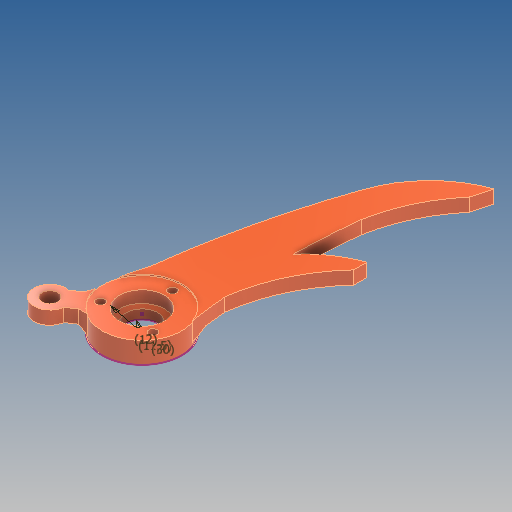
# Autodesk Inventor part: 01-03-01 Zange links nue
Saved by Autodesk Inventor 2026.2 (Build 302298000, 298)
## iProperties
Created: 2025-12-11
Part Number: 01-03-01 Zange links nue
Material: Phenolharz
Document SubType Name: Modeling
Designer: Schally
Density: 1.38 g/cm^3
Appearance: Glatt - Hellorange
Author: Schally
Autodesk Inventor part; units mm, degrees
sketch "Skizze10" plane through (0, 0, 0) normal (1, 0, 0) x (0, 1, 0)
  line L0 (-1.4, 0) -> (8.4, 0) projected
  line L1 (0, -13.2) -> (0, 2.2) projected
  line L2 (2, -2.5) -> (7, -2.5)
  line L3 (7, -2.5) -> (7, -8)
  line L4 (7, -8) -> (2, -8)
  line L5 (2, -8) -> (2, -2.5)
  point P0 (0, 0)
  point P1 (0, -11)
  dimension "d135" = 8
  dimension "d137" = 5
  dimension "d138" = 2
  dimension "d145" = 2.5
  constraints: 8 end point, 2 parallel, 1 horizontal, 1 perpendicular, 1 point on line
  measures "d135" distance between parallel lines of L0 L4
  measures "d137" distance between parallel lines of L5 L3
  measures "d138" distance between parallel lines of L1 L5
  measures "d145" distance between parallel lines of L0 L2
revolve "Umdrehung2" add sketch "Skizze10" angle 360 about axis through (0, -10, 0) along (0, 1, 0)
ref_plane "Arbeitsebene2" through (0, 6, 0) normal (0, 1, 0) x (1, 0, 0)
ref_plane "Arbeitsebene3" through (0, 4.5, 0) normal (0, 1, 0) x (1, 0, 0)
sketch "Skizze12" plane through (0, 4.5, 0) normal (0, 1, 0) x (1, 0, 0)
  arc A0 (3.5, 80) -> (-11.5, 15.25) centre (296.2619, -21.9337) ccw projected
  arc A1 (28, 100) -> (13, 70) centre (72.0267, 59.2367) ccw projected
  line L0 (28, 100) -> (28, 105) projected
  arc A2 (28, 105) -> (3.5, 80) centre (41.4387, 67.3251) ccw projected
  circle A3 centre (0, 0) radius 15
  arc A4 (-11.5, 15.25) -> (-15, 0) centre (120.624, -23.1002) ccw
  circle A5 centre (0, 0) radius 8 projected
  line L1 (0, 0) -> (-20.4788, -14.3394)
  line L2 (-78.9324, 0) -> (358.7942, 0) projected
  line L3 (0, 133.8507) -> (0, -48.3491) projected
  circle A6 centre (-20.4788, -14.3394) radius 6
  circle A7 centre (-20.4788, -14.3394) radius 3
  line L4 (2.2943, -3.2766) -> (-14.5211, -15.0509)
  line L5 (-2.2943, 3.2766) -> (-19.1097, -8.4977)
  arc A8 (28, 52) -> (12.5126, 18.8571) centre (72.0267, 11.2367) ccw
  line L6 (28, 52) -> (28, 57)
  arc A9 (28, 57) -> (11.4602, 45.8069) centre (41.4387, 19.3251) ccw
  arc A10 (13, 70) -> (11.4602, 45.8069) centre (261.1443, 42.0613) ccw
  arc A11 (12.5126, 18.8571) -> (15, 0) centre (261.1443, 42.0613) ccw
  line L7 (28, 105) -> (24.0256, 90.1672)
  point P0 (-16.4, 0)
  point P1 (-14.1366, -5.0155)
  point P2 (-10.4814, -11.4821)
  point P3 (-7.2048, -13.7764)
  point P4 (-9.548, -11.5687)
  point P5 (28, 54.5)
  point P6 (28, 102.5)
  point P7 (-13.9387, 5.5419)
  point P8 (14.2414, 4.7098)
  point P9 (26.0755, 97.8175)
  dimension "d147" = 30
  dimension "d148" = 55
  dimension "d149" = 25
  dimension "d150" = 12
  dimension "d152" = 3
  dimension "d153" = 4
  dimension "d154" = 4
  dimension "d221" = 57
  dimension "d222" = 15
  constraints: 14 point on circle, 10 end point, 8 centre point, 3 coincident, 2 midpoint, 2 parallel, 1 vertical alignment
  measures "d147" diameter of A3
  measures "d148" angle of L1 L3
  measures "d149" distance of L1.start L1.end
  measures "d150" diameter of A6
  measures "d152" radial gap between concentric circles of A6 A7
  measures "d153" distance between parallel lines of L1 L4
  measures "d154" distance between parallel lines of L1 L5
  measures "d221" distance from line of L2 L6.end
  measures "d222" angle of L0 L7
sketch "Skizze13" plane through (0, 4.5, 0) normal (0, 1, 0) x (1, 0, 0)
  point P0 (0, 0)
extrude "Extrusion8" add sketch "Skizze12" along normal mid plane 5 contours A2 L7 A1 A10 A9 L6 A8 A11 A3 L3 A0 | L3 A3 A4 A0 | L3 A5 L2 A4 A3 | A3 A11 L2 A5 L3 | A4 A3 | A3 A11 | L3 L2 A5 | A5 L2 L3 | L2 A5 L5 A3 | A3 L3 A5 L2 | A5 L3 L2 | L2 L5 A5 | L3 L4 A5 L1 | L1 A5 L5 L2 | L5 A5 L1 A3 | A3 L1 A6 L5 | A3 L4 A5 L3 | A5 L4 L3 | A5 L4 A3 L1 | A3 L4 A6 L1 | A6
sketch "Skizze15" plane through (0, 4.5, 0) normal (0, 1, 0) x (1, 0, 0)
  arc A0 (-11.5, 15.25) -> (-13.9387, 5.5419) centre (120.624, -23.1002) ccw projected
  circle A1 centre (0, 0) radius 15
  point P0 (-15, 0)
  constraints: 1 coincident, 1 horizontal alignment, 2 other
extrude "Extrusion10" add sketch "Skizze15" along normal mid plane 12
sketch "Skizze16" plane through (0, 4.5, 0) normal (0, 1, 0) x (1, 0, 0)
  circle A0 centre (0, 0) radius 6
  dimension "d162" = 12
  constraints: 1 centre point, 1 coincident
  measures "d162" diameter of A0
extrude "Extrusion11" cut sketch "Skizze16" along normal mid plane 12
sketch "Skizze17" plane through (0, 4.5, 0) normal (0, 1, 0) x (1, 0, 0)
  circle A0 centre (0, 0) radius 8.5
  dimension "d165" = 17
  constraints: 1 centre point, 1 coincident
  measures "d165" diameter of A0
extrude "Extrusion12" cut sketch "Skizze17" along normal mid plane 5
chamfer "Fasen7" distance 2 angle 45 8 edges at (-12.2873, 7, 8.6036) (-9.548, 3.25, 11.5687) (-9.548, 5.75, 11.5687) (-12.2873, 2, 8.6036) (0.4428, 2, -14.9935) (0.4428, 7, -14.9935) (-14.1366, 5.75, 5.0155) (-14.1366, 3.25, 5.0155)
ref_plane "Arbeitsebene4" through (0, 4.5, 0) normal (0, 1, 0) x (1, 0, 0)
sketch "Skizze21" plane through (0, 10.5, 0) normal (0, 1, 0) x (1, 0, 0)
  circle A0 centre (0, 0) radius 15
  dimension "d200" = 30
  constraints: 1 centre point, 1 coincident
  measures "d200" diameter of A0
extrude "Extrusion16" cut sketch "Skizze21" against normal blind 4
sketch "Skizze23" plane through (0, 6.5, 0) normal (0, 1, 0) x (1, 0, 0)
  line L0 (-37.3746, 0) -> (38.8958, 0) projected
  line L1 (0, 130.102) -> (0, -45.6119) projected
  line L2 (0, 0) -> (0, 20.1991)
  line L3 (0, 0) -> (-17.4929, -10.0995)
  line L4 (0, 0) -> (17.4929, -10.0995)
  circle A0 centre (0, 0) radius 8.5 projected
  arc A1 (14.2414, 4.7098) -> (-13.9387, 5.5419) centre (0, 0) ccw projected
  circle A2 centre (0, 0) radius 11.5
  circle A3 centre (-9.9593, -5.75) radius 1.6
  circle A4 centre (9.9593, -5.75) radius 1.6
  circle A5 centre (0, 11.5) radius 1.6
  arc A6 (-13.9387, 5.5419) -> (-14.6782, -3.0902) centre (0, 0) ccw projected
  arc A7 (-7.9241, -12.7361) -> (14.2414, 4.7098) centre (0, 0) ccw projected
  arc A8 (-14.6782, -3.0902) -> (-7.9241, -12.7361) centre (0, 0) ccw projected
  dimension "d203" = 360
  dimension "d205" = 3
  dimension "d206" = 3.2
  dimension "d207" = 3.2
  dimension "d208" = 3.2
  dimension "d216" = 23
  dimension "d217" = 120
  constraints: 6 end point, 4 centre point, 4 point on line, 3 point on circle, 2 coincident, 8 other
  measures "d205" radial gap between concentric circles of A0 A2
  measures "d206" diameter of A3
  measures "d207" diameter of A4
  measures "d208" diameter of A5
  measures "d216" diameter of A2
  measures "d217" angle of L1 L4
extrude "Extrusion17" cut sketch "Skizze23" against normal blind 8 contours A5 A2 L1 | L1 A2 A5 | A3 A2 L3 | L3 A2 A3 | A4 A2 L4 | L4 A2 A4 | A2 L1 A5 | A4 L4 A2 | A5 L1 A2 | A2 L3 A3 | A3 L3 A2 | A2 L4 A4
sketch "Skizze24" plane through (0, -1.5, 0) normal (0, -1, 0) x (1, 0, 0)
  circle A0 centre (0, -11.5) radius 1.6 projected
  circle A1 centre (9.9593, 5.75) radius 1.6 projected
  circle A2 centre (-9.9593, 5.75) radius 1.6 projected
  circle A3 centre (0, 0) radius 6 projected
  circle A4 centre (0, 0) radius 15 projected
  dimension "d211" = 12
  dimension "d212" = 30
  dimension "d213" = 11.5
  measures "d211" diameter of A3
  measures "d212" diameter of A4
  measures "d213" distance of point (0, 0) A1.centre
sketch "Skizze25" plane through (28, 7, -100) normal (0, 1, 0) x (1, 0, 0)
  line L0 (-56.3412, -125.0488) -> (1.0248, -125.0488)
  line L1 (1.0248, -125.0488) -> (1.0248, -72.2498)
  line L2 (1.0248, -72.2498) -> (-56.3412, -72.2498)
  line L3 (-56.3412, -72.2498) -> (-56.3412, -125.0488)
  constraints: 8 end point, 2 parallel, 1 horizontal, 1 perpendicular
extrude "Extrusion18" cut sketch "Skizze25" along normal blind 10
sketch "Skizze26" plane through (0, -1.5, 0) normal (0, -1, 0) x (1, 0, 0)
  circle A0 centre (0, -11.5) radius 1.6 projected
  circle A1 centre (9.9593, 5.75) radius 1.6 projected
  circle A2 centre (-9.9593, 5.75) radius 1.6 projected
  circle A3 centre (-9.9593, 5.75) radius 2.1
  circle A4 centre (9.9593, 5.75) radius 2.1
  circle A5 centre (0, -11.5) radius 2.1
  dimension "d223" = 4.2
  dimension "d224" = 4.2
  dimension "d225" = 4.2
  constraints: 3 centre point, 3 coincident
  measures "d223" diameter of A3
  measures "d224" diameter of A4
  measures "d225" diameter of A5
extrude "Extrusion19" cut sketch "Skizze26" against normal blind 6 contours A0 | A1 | A2 | A3 | A4 | A5
